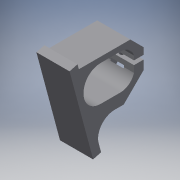
# Autodesk Inventor part: Stand_Front
Saved by Autodesk Inventor 2018 (Build 220112000, 112)
## iProperties
Created: 2018-02-04
Part Number: Stand_Front
Material: Generic
Document SubType Name: Modeling
Designer: Mandus
Density: 1 g/cm^3
Appearance: Default
Author: Mandus
Autodesk Inventor part; units mm, degrees
ref_plane "YZ Plane" through (0, 0, 0) normal (1, 0, 0) x (0, 1, 0)
ref_plane "XZ Plane" through (0, 0, 0) normal (0, 1, 0) x (-1, 0, 0)
ref_plane "XY Plane" through (0, 0, 0) normal (0, 0, 1) x (1, 0, 0)
sketch "Sketch1" plane through (0, 0, 0) normal (0, 0, 1) x (1, 0, 0)
  line L0 (16, 15) -> (95, 15) construction
  line L1 (10, 15) -> (130, 15) construction
  circle A0 centre (34.5, 18) radius 1.5 projected
  circle A1 centre (72.7, 18) radius 1.5 construction
  circle A2 centre (109.5, 18) radius 1.5 construction
  line L2 (101, -15) -> (10, -15) construction
  line L3 (24.5, 15) -> (29.5, 15)
  line L4 (24.5, 15) -> (44.5, 15)
  line L5 (44.5, 15) -> (44.5, 21)
  line L6 (44.5, 21) -> (24.5, 21)
  line L7 (24.5, 21) -> (24.5, 15)
  line L8 (24.5, 15) -> (44.5, 15)
  line L9 (44.5, 15) -> (44.5, -25)
  line L10 (44.5, -25) -> (24.5, -25)
  line L11 (24.5, -25) -> (24.5, 15)
  line L12 (30.5, 15) -> (38.5, 15)
  line L13 (38.5, 15) -> (38.5, -15)
  line L14 (38.5, -15) -> (30.5, -15)
  line L15 (30.5, -15) -> (30.5, 15)
  point P0 (0, 0)
  point P1 (34.5, 21)
  dimension "d9" = 20
  dimension "d10" = 6
  dimension "d16" = 20
  dimension "d17" = 6
  dimension "d18" = 6
  dimension "d19" = 10
  constraints: 26 end point, 6 parallel, 4 horizontal, 3 perpendicular, 2 point on line, 1 horizontal alignment, 1 midpoint, 1 vertical alignment
  measures "d9" distance of L6.end L5.end
  measures "d10" distance of L5.end L4.end
  measures "d16" distance of L9.end L10.end
  measures "d17" distance from line of L15 L3.start
  measures "d18" distance from line of L13 L4.end
  measures "d19" distance from line of L2 L10.end
extrude "Extrusion1" add sketch "Sketch1" along normal blind 12
sketch "Sketch2" plane through (0, 0, 12) normal (0, 0, 1) x (1, 0, 0)
  line L0 (30.5, 15) -> (38.5, 15) projected
  line L1 (30.5, 15) -> (38.5, 15)
  line L2 (38.5, 15) -> (38.5, 21)
  line L3 (38.5, 21) -> (30.5, 21)
  line L4 (30.5, 21) -> (30.5, 15)
  point P0 (0, 0)
  dimension "d22" = 8
  dimension "d23" = 6
  constraints: 8 end point, 2 parallel, 1 horizontal, 1 perpendicular
  measures "d22" distance of L3.end L2.end
  measures "d23" distance of L2.end L1.end
extrude "Extrusion2" cut sketch "Sketch2" against normal blind 9
chamfer "Chamfer1" distance 8 angle 45 2 edges at (41.5, 21, 12) (27.5, 21, 12)
thicken "Thicken1" [suppressed]
sketch "Sketch4" plane through (24.5, -25, 0) normal (-1, 0, 0) x (0, 0, 1)
  line L0 (14.998863, 6.117714) -> (0.509975, 10)
  line L1 (0.509975, 10) -> (-38.127058, 20.352762)
  line L2 (12, 38) -> (12, 0)
  line L3 (12, 6.921257) -> (12, 0)
  line L4 (12, 0) -> (0, 0)
  line L5 (0, 46) -> (0, 0)
  line L6 (0, 0) -> (0, 9.910897)
  arc A0 (0, 9.910897) -> (8.7, 20) centre (-1.5, 20) ccw
  point P0 (0, 25)
  constraints: 6 end point, 2 perpendicular, 2 point on line, 1 collinear
extrude "Extrusion4" cut sketch "Sketch4" against normal up to next contours L2 L4 L5 A0 L0
sketch "Sketch6" plane through (24.5, 21, 0) normal (-1, 0, 0) x (0, 0, 1)
  line L0 (-20, -12) -> (-8, 0)
  line L1 (-20, -12) -> (-20, -17.472115)
  arc A0 (-32.58819, -27.131373) -> (-20, -17.472115) centre (-30, -17.472115) ccw
  line L2 (-32.58819, -27.131373) -> (-38.127058, -25.647238)
  line L3 (-38.127058, -25.647238) -> (-39.421153, -30.476867)
  line L4 (-39.421153, -30.476867) -> (13.704767, -44.711915)
  line L5 (13.704767, -44.711915) -> (14.998863, -39.882286)
  line L6 (14.998863, -39.882286) -> (-2.5, -35.19348)
  line L7 (-2.5, -35.19348) -> (-2.5, 0)
  line L8 (-2.5, 0) -> (-8, 0)
  point P0 (0, -21)
extrude "Extrusion6" add sketch "Sketch6" against normal up to surface (20 mm away)
sketch "Sketch7" plane through (24.5, 21, 0) normal (-1, 0, 0) x (0, 0, 1)
  spline S0 degree 3 poles (-6.5, -6) (-6.546693, -6.013254) (-6.616732, -6.033135) (-6.941908, -6.140497) (-7.152984, -6.216066) (-7.849197, -6.507561) (-8.38978, -6.791544) (-9.381679, -7.471651) (-9.918841, -7.925952) (-10.890727, -9.023195) (-11.3248, -9.667651) (-11.895906, -10.836743) (-12.110628, -11.410204) (-12.256441, -12) knots 0 0 0 0 0.11327255 0.11327255 0.2265451 0.2265451 0.45309019 0.45309019 0.68571665 0.68571665 0.9183431 0.9183431 1.08886769 1.08886769 1.08886769 1.08886769
  line L0 (2.5, -6) -> (-6.5, -6)
  spline S1 degree 3 poles (8.256441, -12) (8.038052, -11.116642) (7.660143, -10.245909) (6.692123, -8.740362) (6.10323, -8.10388) (4.935072, -7.121845) (4.264812, -6.714774) (3.37825, -6.3035) (3.105893, -6.198836) (2.780187, -6.086268) (2.686062, -6.056295) (2.546182, -6.013279) (2.518473, -6.005312) (2.5, -6) knots -1.11087633 -1.11087633 -1.11087633 -1.11087633 -0.83789048 -0.83789048 -0.56490462 -0.56490462 -0.28245231 -0.28245231 -0.14122616 -0.14122616 -0.07061308 -0.07061308 0 0 0 0
  arc A0 (8.5, -14) -> (8.256441, -12) centre (0.166667, -14) ccw
  line L1 (8.5, -26) -> (8.5, -14)
  arc A1 (-1.5, -36) -> (8.5, -26) centre (-1.5, -26) ccw
  arc A2 (-12.5, -26) -> (-2.5, -36) centre (-2.5, -26) ccw
  line L2 (-12.5, -14) -> (-12.5, -26)
  arc A3 (-12.256441, -12) -> (-12.5, -14) centre (-4.166667, -14) ccw
  line L3 (-2.5, -36) -> (-1.5, -36)
  point P0 (0, -21)
extrude "Extrusion7" cut sketch "Sketch7" against normal up to surface (20 mm away)
thicken "Thicken2" operation add thickness 0.2 both sides no extend neighbours yes toward (0, 1, 0) faces at (31.166667, 15, -3.833333) (34.5, 10.333301, -11.803914) (37.833333, 7.224386, -12.496979) (31.166667, 3, -12.5) (37.833333, -14.972038, -3.247301) (31.166667, -15, -2.166667) (37.833333, -10, 7.160254) (31.166667, -1, 8.5) (37.833333, 8.118677, 8.424572) (34.5, 10.718673, 7.622797) (31.166667, 15, 1.666667)
sketch "Sketch8" plane through (24.5, 21, -2.5) normal (0, 1, 0) x (1, 0, 0)
  line L0 (14, -5.5) -> (6, -5.5) construction
  line L1 (6, -5.5) -> (6, 19.5) construction
  line L2 (6, 19.5) -> (14, 19.5) construction
  line L3 (14, 19.5) -> (14, -5.5) construction
  line L4 (14, 19.5) -> (6, 19.5)
  line L5 (6, 19.5) -> (6, 3)
  line L6 (6, 3) -> (14, 3)
  line L7 (14, 3) -> (14, 19.5)
  point P0 (-24.5, -2.5)
  dimension "d44" = 8
  dimension "d45" = 25
  dimension "d46" = 8
  dimension "d47" = 16.5
  constraints: 16 end point, 4 parallel, 2 horizontal, 2 perpendicular
  measures "d44" distance of L1.end L2.end
  measures "d45" distance of L0.end L1.end
  measures "d46" distance of L6.end L5.end
  measures "d47" distance of L5.end L4.end
extrude "Extrusion8" cut sketch "Sketch8" against normal up to surface (6 mm away)
sketch "Sketch9" plane through (0, 0, 3) normal (0, 0, 1) x (1, 0, 0)
  circle A0 centre (34.5, 18) radius 1.5 projected
  point P0 (0, 0)
extrude "Extrusion9" cut sketch "Sketch9" against normal up to surface (8.5 mm away)
body "Solid1"
